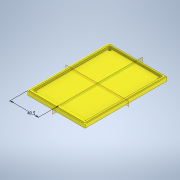
# Autodesk Inventor part: top
Saved by Autodesk Inventor 2022.2 (Build 262287000, 287)
## iProperties
Created: 2021-12-01
Part Number: top
Material: Generic
Document SubType Name: Modeling
Designer: samlo
Density: 1 g/cm^3
Appearance: Canary
Author: samlo
Autodesk Inventor part; units mm, degrees
ref_plane "YZ Plane" through (0, 0, 0) normal (1, 0, 0) x (0, 1, 0)
ref_plane "XZ Plane" through (0, 0, 0) normal (0, 1, 0) x (-1, 0, 0)
ref_plane "XY Plane" through (0, 0, 0) normal (0, 0, 1) x (1, 0, 0)
sketch "Sketch1" plane through (0, 0, 0) normal (0, 1, 0) x (-1, 0, 0)
  line L0 (0, 0) -> (81, 0)
  line L1 (81, 0) -> (81, -116)
  line L2 (81, -116) -> (0, -116)
  line L3 (0, -116) -> (0, 0)
  dimension "d0" = 116
  dimension "d1" = 81
  constraints: 8 end point, 2 parallel, 1 horizontal, 1 perpendicular
  measures "d0" distance of L2.end L0.start
  measures "d1" distance of L0.start L0.end
extrude "Extrusion1" add sketch "Sketch1" along normal blind 3
sketch "Sketch2" plane through (0, 3, 0) normal (0, 1, 0) x (1, 0, 0)
  line L0 (0, 116) -> (-81, 116) projected
  line L1 (0, 0) -> (-81, 0)
  line L2 (-81, 0) -> (-81, 116)
  line L3 (-81, 116) -> (0, 116)
  line L4 (0, 116) -> (0, 0)
  line L5 (-3, 3) -> (-78, 3)
  line L6 (-78, 3) -> (-78, 113)
  line L7 (-78, 113) -> (-3, 113)
  line L8 (-3, 113) -> (-3, 3)
  dimension "d8" = 75
  dimension "d9" = 110
  dimension "d10" = 3
  dimension "d11" = 3
  constraints: 16 end point, 4 parallel, 2 horizontal, 2 perpendicular
  measures "d8" distance of L5.start L5.end
  measures "d9" distance of L7.end L5.start
  measures "d10" horizontal distance of L5.start L1.start
  measures "d11" horizontal distance of L5.start L1.start
extrude "Extrusion2" add sketch "Sketch2" along normal blind 3
sketch "Sketch3" plane through (0, 6, 0) normal (0, 1, 0) x (1, 0, 0)
  line L0 (-78, 3) -> (-3, 3) projected
  line L1 (-40.5, 0) -> (-40.5, 3)
  line L2 (-81, 116) -> (-81, 0) projected
  point P0 (0, 0)
  point P1 (-40.5, 1.5)
  dimension "d18" = 40.5
  constraints: 2 end point, 2 midpoint, 1 vertical
  measures "d18" distance from line of point (-40.5, 1.5) L2
lip "Lip1" kind groove height 1 width 1 edges at (-40.5, 6, 0) (0, 6, -58) (-40.5, 6, -116) (-81, 6, -58) guide face at (-80, 6, -76.3333)
sketch "Sketch4" plane through (0, 3, 0) normal (0, 1, 0) x (1, 0, 0)
  circle A0 centre (-5.5, 5.5) radius 1.5
  line L0 (-3, 3) -> (-78, 3) projected
  line L1 (-3, 113) -> (-3, 3) projected
  point P0 (0, 0)
  dimension "d27" = 3
  dimension "d28" = 2.5
  dimension "d29" = 2.5
  constraints: 1 centre point
  measures "d27" diameter of A0
  measures "d28" distance from line of A0.centre L0
  measures "d29" distance from line of L1 A0.centre
extrude "Extrusion3" cut sketch "Sketch4" against normal through all
ref_plane "Work Plane1" through (-81, 0, -58) normal (0, 0, 1) x (1, 0, 0)
ref_plane "Work Plane2" through (-40.5, 0, -116) normal (-1, 0, 0) x (0, 0, 1)
mirror "Mirror1" about plane through (-81, 0, -58) normal (0, 0, 1) of "Extrusion3"
mirror "Mirror2" about plane through (-40.5, 0, -116) normal (-1, 0, 0) of "Extrusion3"
mirror "Mirror3" about plane through (-81, 0, -58) normal (0, 0, 1) of "Extrusion3", "Mirror2"
body "Solid1"
